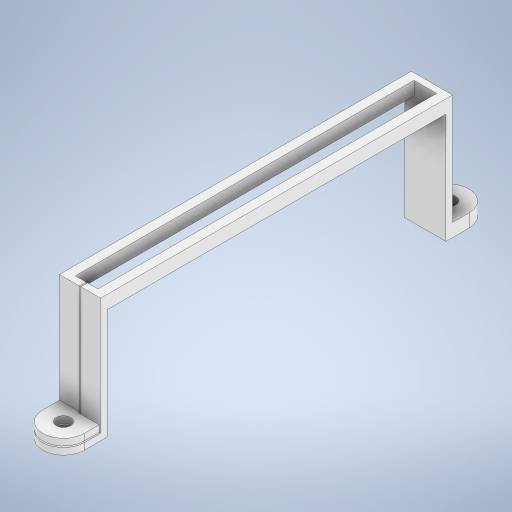
# Autodesk Inventor part: WIRE_HOUSING
Saved by Autodesk Inventor 2023 (Build 270158000, 158)
## iProperties
Created: 2023-03-21
Part Number: WIRE_HOUSING
Material: PC/ABS Plastic
Document SubType Name: Modeling
Designer: Amos Yu
Density: 0.357273 g/cm^3
Appearance: White
Author: Amos Yu
Autodesk Inventor part; units mm, degrees
ref_plane "YZ Plane" through (0, 0, 0) normal (1, 0, 0) x (0, 1, 0)
ref_plane "XZ Plane" through (0, 0, 0) normal (0, 1, 0) x (-1, 0, 0)
sketch "Sketch1" plane through (0, 0, 0) normal (0, 1, 0) x (-1, 0, 0)
  circle A0 centre (0, 0) radius 1.1
  arc A1 (3.1, 0) -> (-3.1, 0) centre (0, 0) ccw
  circle A2 centre (0, -58) radius 1.1
  arc A3 (-3.1, -58) -> (3.1, -58) centre (0, -58) ccw
  line L0 (3.1, -58) -> (3.1, -54.5)
  line L1 (-3.1, -58) -> (-3.1, -54.5)
  line L2 (3.1, -54.5) -> (-3.1, -54.5)
  line L3 (3.1, -3.5) -> (-3.1, -3.5)
  line L4 (-3.1, -3.5) -> (-3.1, 0)
  line L5 (3.1, 0) -> (3.1, -3.5)
  line L6 (3.1, -55.5) -> (-3.1, -55.5)
  line L7 (3.1, -2.5) -> (-3.1, -2.5)
  line L8 (-0.1, -2.5) -> (-0.1, -3.5)
  dimension "d0" = 2.2
  dimension "d1" = 2
  dimension "d2" = 2.2
  dimension "d3" = 2
  dimension "d4" = 58
  dimension "d5" = 3.5
  dimension "d6" = 3.5
  dimension "d7" = 1
  dimension "d8" = 1
  dimension "d17" = 0.1
  constraints: 18 end point, 6 point on line, 4 centre point, 4 perpendicular, 4 point on circle, 4 tangent, 3 coincident, 2 horizontal, 2 parallel, 2 vertical, 1 vertical alignment
  measures "d0" diameter of A0
  measures "d1" radial gap between concentric circles of A1 A0
  measures "d2" diameter of A2
  measures "d3" radial gap between concentric circles of A2 A3
  measures "d4" distance of A2.centre point (0, 0)
  measures "d5" distance of L0.start L0.end
  measures "d6" distance of L3.end L4.end
  measures "d7" distance between parallel lines of L2 L6
  measures "d8" distance between parallel lines of L3 L7
  measures "d17" distance from line of point (0, 0) L8
extrude "Extrusion1" add sketch "Sketch1" along normal blind 2 contours L1 L6 L0 A3
extrude "Extrusion5" add sketch "Sketch1" along normal blind 1 contours L5 L7 L4 A1 | L5 L3 L8 L7
extrude "Extrusion2" add sketch "Sketch1" along normal blind 16.6 contours L7 L8 L3 L4 | L1 L2 L0 L6
sketch "Sketch2" plane through (0, 16.6, 0) normal (0, 1, 0) x (1, 0, 0)
  line L0 (-3.1, 2.5) -> (-3.1, 0) construction
  line L1 (3.1, 55.5) -> (3.1, 58) construction
  line L2 (-3.1, 2.5) -> (3.1, 2.5)
  line L3 (3.1, 2.5) -> (3.1, 55.5)
  line L4 (3.1, 55.5) -> (-3.1, 55.5)
  line L5 (-3.1, 55.5) -> (-3.1, 2.5)
  line L6 (3.1, 3.5) -> (0.1, 3.5) construction
  line L7 (-3.1, 54.5) -> (3.1, 54.5) construction
  line L8 (-1.7, 3.5) -> (1.7, 3.5)
  line L9 (1.7, 3.5) -> (1.7, 54.5)
  line L10 (1.7, 54.5) -> (-1.7, 54.5)
  line L11 (-1.7, 54.5) -> (-1.7, 3.5)
  line L12 (3.1, 3.5) -> (-3.1, 3.5) projected
  line L13 (-0.1, 3.5) -> (-0.1, 2.5)
  line L14 (0.1, 3.5) -> (0.1, 2.5)
  point P0 (0, 0)
  point P1 (0, 3.5)
  dimension "d13" = 1.4
  dimension "d14" = 1.4
  dimension "d37" = 0.2
  dimension "d38" = 0.1
  constraints: 20 end point, 6 point on line, 4 parallel, 4 perpendicular, 2 horizontal, 1 midpoint
  measures "d13" distance between parallel lines of L5 L11
  measures "d14" distance between parallel lines of L9 L3
  measures "d37" distance between parallel lines of L13 L14
  measures "d38" distance from line of L14 point (0, 3.5)
extrude "Extrusion3" add sketch "Sketch2" along normal blind 2 contours L5 L12 L8 L13 L2 | L5 L4 L3 L12 L9 L10 L11 | L14 L8 L12 L3 L2
ref_plane "Work Plane3" through (0, 1.2, 0) normal (0, 1, 0) x (1, 0, 0)
sketch "Sketch4" plane through (0, 1.2, 0) normal (0, 1, 0) x (1, 0, 0)
  arc A0 (-3.1, 0) -> (3.1, 0) centre (0, 0) ccw projected
  circle A1 centre (0, 0) radius 1.1 projected
  line L0 (-3.1, 3.5) -> (-3.1, 0) construction
  line L1 (3.1, 0) -> (3.1, 3.5) construction
  line L2 (3.1, 2.3) -> (3.1, 0)
  line L3 (3.1, 2.5) -> (0.1, 2.5) construction
  line L4 (-0.1, 2.3) -> (-0.1, 3.5)
  line L5 (-0.1, 3.5) -> (-3.1, 3.5)
  line L6 (3.1, 2.5) -> (0.1, 2.5) projected
  line L7 (-3.1, 2.5) -> (-0.1, 2.5)
  line L8 (-0.1, 2.3) -> (3.1, 2.3)
  line L9 (-3.1, 0) -> (-3.1, 3.5)
  dimension "d28" = 0.1
  dimension "d29" = 1
  dimension "d30" = 0.2
  constraints: 12 end point, 2 perpendicular, 2 point on line, 1 collinear, 1 vertical
  measures "d28" distance from line of point (0, 0) L4
  measures "d29" distance between parallel lines of L3 L5
  measures "d30" distance between parallel lines of L3 L8
extrude "Extrusion6" add sketch "Sketch4" along normal blind 1
extrude "Extrusion8" add sketch "Sketch4" along normal up to surface (15.4 mm away) contours L9 L5 L4 L7
equation "\"d0\" = bolt_thread_diameter + 2 * tol"
equation "\"d1\" = thickness"
equation "\"d2\" = bolt_thread_diameter + 2 * tol"
equation "\"d3\" = thickness"
equation "\"d4\" = hole_separation"
equation "\"d5\" = hole_pin_separation - tol"
equation "\"d6\" = hole_pin_separation - tol"
equation "\"d7\" = minor_thickness"
equation "\"d8\" = minor_thickness"
equation "\"d17\" = tol"
equation "\"d9\" = thickness"
equation "\"d24\" = 0.5 * thickness"
equation "\"d11\" = wire_height + pin_base_height + tol"
equation "\"d13\" = overhang"
equation "\"d14\" = overhang"
equation "\"d37\" = 2 * tol"
equation "\"d38\" = tol"
equation "\"d15\" = thickness"
equation "\"d28\" = tol"
equation "\"d29\" = minor_thickness"
equation "\"d30\" = 2 * tol"
equation "\"d31\" = 0.5 * thickness"
equation "\"d35\" = 0.5 * thickness"
equation "\"wire_height\" = 14"
equation "\"hole_separation\" = 58"
equation "\"pin_base_height\" = 2.5"
equation "\"hole_pin_separation\" = 3.6"
equation "\"minor_thickness\" = 1"
equation "\"overhang\" = 1.4"
equation "\"d26\" = 2 * tol"
equation "\"bolt_thread_diameter\" = 2"
equation "\"tol\" = 0.1"
equation "\"thickness\" = 2"
body "Solid1"
